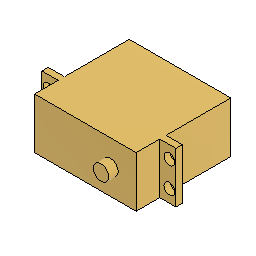
M-side assembly V2 v15 (Autodesk Fusion 360 archive; units mm, degrees)
design "HS-322HD"
Autodesk Fusion 360 part; units mm, degrees
sketch "스케치1" plane through (0, 0, 0) normal (0, 0, 1) x (1, 0, 0)
  line L0 (0, 0) -> (40, 0)
  line L1 (40, 0) -> (40, 36.5)
  line L2 (40, 36.5) -> (0, 36.5)
  line L3 (0, 36.5) -> (0, 0)
  dimension "d1" = 40
  dimension "d2" = 36.5
  constraint horizontal L0
  constraint vertical L1
  constraint horizontal L2
  constraint vertical L3
  constraint coincident L0.start L3.end
  measures "d1" distance of L0.start L0.end
  measures "d2" distance of L0.start L2.end
extrude "돌출1" add sketch "스케치1" along normal blind 20
sketch "스케치2" plane through (0, 36.5, 0) normal (0, 1, 0) x (-1, 0, 0)
  line L0 (-40, 0) -> (0, 0)
  line L1 (0, 0) -> (0, 20)
  line L2 (0, 20) -> (-40, 20)
  line L3 (-40, 20) -> (-40, 0)
  line L4 (-20, 20) -> (6.4, 20)
  line L5 (6.4, 20) -> (6.4, 0)
  line L6 (6.4, 0) -> (-20, 0)
  line L7 (-20, 20) -> (-20, 0)
  line L8 (-46.4, 0) -> (-20, 0)
  line L9 (-46.4, 20) -> (-46.4, 0)
  line L10 (-20, 20) -> (-46.4, 20)
  circle A0 centre (3.8, 15.05) radius 2.15
  circle A1 centre (3.8, 4.95) radius 2.15
  line L11 (6.4, 10) -> (-20, 10)
  line L12 (3.8, 15.05) -> (3.8, 20)
  line L13 (3.8, 4.95) -> (3.8, 0)
  circle A2 centre (-43.8, 4.95) radius 2.15
  circle A3 centre (-43.8, 15.05) radius 2.15
  circle A4 centre (-29.9, 10) radius 3
  line L14 (-29.9, 10) -> (-20, 10)
  dimension "d5" = 26.4
  dimension "d6" = 4.3
  dimension "d7" = 4.3
  dimension "d8" = 10.1
  dimension "d9" = 4.95
  dimension "d10" = 4.95
  dimension "d11" = 23.8
  dimension "d12" = 16.5
  constraint midpoint L2 L4.start
  constraint perpendicular L1 L4
  constraint perpendicular L4 L5
  constraint midpoint L0 L6.end
  constraint perpendicular L1 L6
  constraint symmetric L4.start L7 L10.start
  constraint symmetric L4.end L7 L9.start
  constraint symmetric L5.end L7 L8.start
  constraint symmetric L6.end L7 L8.end
  constraint midpoint L5 L11.start
  constraint midpoint L7 L11.end
  constraint coincident A0.centre L12.start
  constraint coincident L4 L12.end
  constraint perpendicular L4 L12
  constraint coincident A1.centre L13.start
  constraint coincident L6 L13.end
  constraint perpendicular L6 L13
  constraint symmetric L7 A0 A3
  constraint symmetric L7 A1 A2
  constraint coincident A4.centre L14.start
  measures "d5" distance of L4.start L4.end
  measures "d6" diameter of A0
  measures "d7" diameter of A1
  measures "d8" distance of A0.centre A1.centre
  measures "d9" distance of L4 A0.centre
  measures "d10" distance of L6 A1.centre
  measures "d11" distance of L7 A0.centre
  measures "d12" distance of L9 A4.centre
extrude "돌출2" add sketch "스케치2" against normal blind 36.5 contours L3 L8 L9 L10 | L1 L5 L6 L11 | L1 L4 L5 L11
extrude "돌출3" cut sketch "스케치2" against normal blind 26.5 contours L3 L8 L9 L10 | L1 L5 L6 L11 | L1 L4 L5 L11
sketch "스케치3" plane through (0, 0, 0) normal (0, -1, 0) x (1, 0, 0)
  circle A0 centre (43.8, 15.05) radius 2.15
  circle A1 centre (43.8, 4.95) radius 2.15
  circle A2 centre (-3.8, 4.95) radius 2.15
  circle A3 centre (-3.8, 15.05) radius 2.15
  line L0 (-6.4, 0) -> (46.4, 0)
  line L1 (46.4, 0) -> (46.4, 20)
  line L2 (46.4, 20) -> (-6.4, 20)
  line L3 (-6.4, 20) -> (-6.4, 0)
  circle A4 centre (43.8, 4.95) radius 2.15
  circle A5 centre (43.8, 15.05) radius 2.15
  line L4 (46.4, 20) -> (46.4, 0)
  line L5 (46.4, 0) -> (40, 0)
  line L6 (40, 0) -> (40, 20)
  line L7 (40, 20) -> (46.4, 20)
  circle A6 centre (-3.8, 4.95) radius 2.15
  circle A7 centre (-3.8, 15.05) radius 2.15
  line L8 (-6.4, 0) -> (-6.4, 20)
  line L9 (-6.4, 20) -> (0, 20)
  line L10 (0, 20) -> (0, 0)
  line L11 (0, 0) -> (-6.4, 0)
extrude "돌출4" cut sketch "스케치3" against normal blind 7.5 contours L0 L2 L3 L8 L9 L10 L11 | L0 L1 L2 L4 L5 L6 L7
sketch "스케치4" plane through (0, 0, 0) normal (0, -1, 0) x (1, 0, 0)
  line L0 (0, 20) -> (0, 0)
  line L1 (0, 0) -> (40, 0)
  line L2 (40, 0) -> (40, 20)
  line L3 (40, 20) -> (0, 20)
  circle A0 centre (29.9, 10) radius 3
  line L4 (46.4, 20) -> (46.4, 0)
  dimension "d19" = 6
  dimension "d21" = 16.5
  measures "d19" diameter of A0
  measures "d21" distance of A0.centre L4
extrude "돌출5" add sketch "스케치4" along normal blind 1.8
extrude "돌출6" add 1 faces at (30.3424, 0, 9.3862) along direction (0, -1, 0) blind 20
extrude "돌출7" cut 1 faces at (30.3424, -20, 9.3862) along direction (0, 1, 0) blind 14.5
extrude "돌출8" cut 1 faces at (26.6667, 36.5, 6.6667) along direction (0, -1, 0) blind 1
equation "d5 = ( 52.8 / 2 ) * 1 mm"
